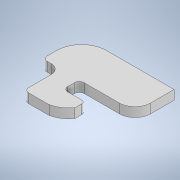
# Autodesk Inventor part: Pi_mount_newupper
Saved by Autodesk Inventor 2022 (Build 260153000, 153)
## iProperties
Created: 2023-02-14
Part Number: Pi_mount_newupper
Material: Generic
Document SubType Name: Modeling
Designer: scott
Density: 1 g/cm^3
Appearance: Default
Author: scott
Autodesk Inventor part; units mm, degrees
ref_plane "YZ Plane" through (0, 0, 0) normal (1, 0, 0) x (0, 1, 0)
ref_plane "XZ Plane" through (0, 0, 0) normal (0, 1, 0) x (-1, 0, 0)
ref_plane "XY Plane" through (0, 0, 0) normal (0, 0, 1) x (1, 0, 0)
sketch "Sketch1" plane through (0, 0, 0) normal (0, 1, 0) x (-1, 0, 0)
  line L0 (0, 0) -> (29.6, 0)
  line L1 (29.6, 0) -> (29.6, 24.2)
  line L2 (29.6, 24.2) -> (0, 24.2)
  line L3 (0, 24.2) -> (0, 0)
  line L4 (29.6, 12.5) -> (0, 12.5)
  line L5 (0, 12.5) -> (0, 0)
  line L6 (0, 0) -> (29.6, 0)
  line L7 (29.6, 0) -> (29.6, 12.5)
  line L8 (23.8, 24.2) -> (10.8, 24.2)
  line L9 (10.8, 24.2) -> (10.8, 12.5)
  line L10 (10.8, 12.5) -> (23.8, 12.5)
  line L11 (23.8, 12.5) -> (23.8, 24.2)
  line L12 (23.8, 17.7) -> (17.8, 17.7)
  line L13 (17.8, 17.7) -> (17.8, 12.5)
  line L14 (17.8, 12.5) -> (23.8, 12.5)
  line L15 (23.8, 12.5) -> (23.8, 17.7)
  line L16 (17.8, 17.7) -> (10.8, 17.7)
  line L17 (10.8, 17.7) -> (10.8, 12.5)
  line L18 (10.8, 12.5) -> (17.8, 12.5)
  line L19 (17.8, 12.5) -> (17.8, 17.7)
  circle A0 centre (21.6, 8) radius 8
  circle A1 centre (5, 7.5) radius 5
  circle A2 centre (16.3, 14) radius 1.5
  circle A3 centre (16.3, 16.2) radius 1.5
  circle A4 centre (26.8, 15.5) radius 3
  circle A5 centre (22.3, 22.7) radius 1.5
  circle A6 centre (11.8, 18.7) radius 1
  line L20 (10.8, 24.2) -> (15.8, 24.2)
  line L21 (15.8, 24.2) -> (15.8, 20.95)
  line L22 (15.8, 20.95) -> (10.8, 20.95)
  line L23 (10.8, 20.95) -> (10.8, 24.2)
  arc A7 (15.8, 24.2) -> (10.8, 20.95) centre (17.6697, 15.8525) ccw
  circle A8 centre (28.1, 11) radius 1.5
  point P0 (17.8, 14)
  point P1 (16.3, 12.5)
  point P2 (5, 12.5)
  point P3 (0, 7.5)
  point P4 (21.6, 0)
  point P5 (29.6, 8)
  point P6 (26.8, 12.5)
  point P7 (23.8, 15.5)
  point P8 (23.8, 22.7)
  point P9 (22.3, 24.2)
  point P10 (10.8, 18.7)
  point P11 (11.8, 17.7)
  point P12 (16.3, 17.7)
  point P13 (17.8, 16.2)
  point P14 (29.6, 11)
  point P15 (28.1, 12.5)
  dimension "d0" = 24.2
  dimension "d1" = 29.6
  dimension "d2" = 11.7
  dimension "d3" = 5.8
  dimension "d4" = 13
  dimension "d5" = 6.5
  dimension "d6" = 6
  dimension "d7" = 16
  dimension "d8" = 8
  dimension "d9" = 8
  dimension "d10" = 10
  dimension "d11" = 5
  dimension "d12" = 5
  dimension "d13" = 3
  dimension "d14" = 3
  dimension "d15" = 1.5
  dimension "d16" = 1.5
  dimension "d17" = 1.5
  dimension "d18" = 1.5
  dimension "d19" = 6
  dimension "d20" = 3
  dimension "d21" = 3
  dimension "d23" = 1.5
  dimension "d24" = 1.5
  dimension "d25" = 2
  dimension "d26" = 1
  dimension "d27" = 1
  dimension "d28" = 5
  dimension "d29" = 3.25
  dimension "d32" = 3
  dimension "d33" = 1.5
  dimension "d34" = 1.5
  dimension "d35" = 12.5
  dimension "d36" = 3
  constraints: 48 end point, 12 parallel, 9 centre point, 6 horizontal, 6 perpendicular, 5 point on line, 2 point on circle
  measures "d0" distance of L0.end L1.end
  measures "d1" distance of L1.end L2.end
  measures "d2" distance between parallel lines of L4 L2
  measures "d3" distance between parallel lines of L1 L11
  measures "d4" distance between parallel lines of L9 L11
  measures "d5" distance between parallel lines of L8 L12
  measures "d6" distance of L12.start L12.end
  measures "d7" diameter of A0
  measures "d8" distance from line of A0.centre L7
  measures "d9" distance from line of L0 A0.centre
  measures "d10" diameter of A1
  measures "d11" distance from line of L4 A1.centre
  measures "d12" distance from line of L3 A1.centre
  measures "d13" diameter of A2
  measures "d14" diameter of A3
  measures "d15" distance from line of L18 A2.centre
  measures "d16" distance from line of L13 A2.centre
  measures "d17" distance from line of L13 A3.centre
  measures "d18" distance from line of L16 A3.centre
  measures "d19" diameter of A4
  measures "d20" diameter of A5
  measures "d21" distance from line of L4 A4.centre
  measures "d23" distance from line of L11 A5.centre
  measures "d24" distance from line of L2 A5.centre
  measures "d25" diameter of A6
  measures "d26" distance from line of L9 A6.centre
  measures "d27" distance from line of L16 A6.centre
  measures "d28" distance of L21.end L22.end
  measures "d29" distance of L20.end L21.end
  measures "d32" diameter of A8
  measures "d33" distance from line of A8.centre L7
  measures "d34" distance from line of L4 A8.centre
  measures "d35" distance between parallel lines of L6 L4
  measures "d36" distance from line of A4.centre L11
extrude "Extrusion1" add sketch "Sketch1" along normal blind 3 contours L3 A1 L4 A0 L0 | A0 L4 A8 | A1 | A0 A8 L1 | A2 L13 L4 | A8 A0 | A8 A0 | L13 A0 L11 L4 | L11 A4 L4 | L13 L12 L11 A0 | L9 L22 L21 L2 A5 L11 L12 L16 A6 | A6 | L16 L13 A3 | L21 L22 A7 | A5 picked at (19.8309, 8.6369)
body "Solid1"
